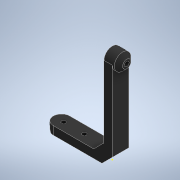
# Autodesk Inventor part: LinearActuatorToBottomPlateAdapter
Saved by Autodesk Inventor 2021 (Build 250183000, 183)
## iProperties
Created: 2020-07-16
Part Number: LinearActuatorToBottomPlateAdapter
Material: Generic
Document SubType Name: Modeling
Designer: CASE-SMALL2
Density: 1 g/cm^3
Appearance: Default
Author: CASE-SMALL2
## iProperties of the stored document _3DPrint.ipt
Created: 2020-07-17
Part Number: _3DPrint
Material: Generic
Document SubType Name: Modeling
Designer: CASE-SMALL2
Density: 1 g/cm^3
Appearance: Default
Author: CASE-SMALL2
Autodesk Inventor part; units mm, degrees
ref_plane "YZ Plane" through (0, 0, 0) normal (1, 0, 0) x (0, 1, 0)
ref_plane "XZ Plane" through (0, 0, 0) normal (0, 1, 0) x (-1, 0, 0)
ref_plane "XY Plane" through (0, 0, 0) normal (0, 0, 1) x (1, 0, 0)
sketch "Sketch3" plane through (0, 0, 0) normal (0, 0, 1) x (1, 0, 0)
  line L0 (0, 0) -> (65, 0)
  line L1 (65, 0) -> (65, 95)
  line L2 (65, 95) -> (57, 95)
  line L3 (57, 95) -> (57, 8)
  line L4 (57, 8) -> (0, 8)
  line L5 (0, 8) -> (0, 0)
  dimension "d17" = 8
  dimension "d18" = 57
  dimension "d19" = 87
  dimension "d20" = 8
  constraints: 12 end point, 5 perpendicular, 1 horizontal
  measures "d17" distance between parallel lines of L4 L0
  measures "d18" distance between parallel lines of L3 L5
  measures "d19" distance between parallel lines of L2 L4
  measures "d20" distance between parallel lines of L3 L1
extrude "Extrusion3" add sketch "Sketch3" against normal mid plane 16
sketch "Sketch5" plane through (0, 8, -8) normal (0, 1, 0) x (1, 0, 0)
  line L0 (-13, -8) -> (78, -8) projected
  circle A0 centre (10, -8) radius 1.9
  circle A1 centre (30, -8) radius 1.9
  line L1 (0, 0) -> (0, -16) projected
  point P0 (0, -8)
  dimension "d23" = 3.8
  dimension "d24" = 3.8
  dimension "d25" = 10
  dimension "d26" = 20
  constraints: 2 centre point, 2 point on line
  measures "d23" diameter of A0
  measures "d24" diameter of A1
  measures "d25" distance from line of L1 A0.centre
  measures "d26" distance of A0.centre A1.centre
extrude "Extrusion4" cut sketch "Sketch5" against normal through all
chamfer "Chamfer2" distance 5 angle 45 1 edges at (0, 0, 0)
chamfer "Chamfer3" distance 10 angle 45 1 edges at (57, 8, 0)
chamfer "Chamfer4" distance 10 angle 45 1 edges at (65, 0, 0)
sketch "Sketch6" plane through (65, 95, 8) normal (1, 0, 0) x (0, 0, -1)
  line L0 (16, -77) -> (16, 0) projected
  line L1 (0, -85) -> (0, 0) projected
  circle A0 centre (8, -8) radius 8
  line L2 (16, 0) -> (0, 0) projected
  point P0 (8, -95)
  dimension "d39" = 16
  constraints: 3 tangent, 1 centre point
  measures "d39" distance between parallel lines of L1 L0
extrude "Extrusion5" add sketch "Sketch6" along normal blind 7 contours A0
fillet "Fillet1" radius 8 2 edges at (61, 95, -8) (61, 95, 8)
sketch "Sketch7" plane through (57, 18, -8) normal (-1, 0, 0) x (0, 0, 1)
  point P0 (8, -18)
sketch "Sketch8" plane through (72, 87, 0) normal (1, 0, 0) x (0, 0, -1)
  circle A0 centre (0, 0) radius 8 projected
  circle A1 centre (0, 0) radius 2.75
  point P0 (0, -87)
  dimension "d43" = 5.5
  constraints: 1 centre point, 1 coincident
  measures "d43" diameter of A1
extrude "Extrusion6" add sketch "Sketch8" along normal blind 4 contours A1
sketch "Sketch9" plane through (76, 87, 0) normal (1, 0, 0) x (0, 0, -1)
  circle A0 centre (0, 0) radius 2.75 construction
  circle A1 centre (0, 0) radius 2.25
  point P0 (0, -87)
  dimension "d46" = 4.5
  constraints: 1 centre point
  measures "d46" diameter of A1
extrude "Extrusion7" cut sketch "Sketch9" against normal through all
sketch "Sketch10" plane through (57, 18, -8) normal (-1, 0, 0) x (0, 0, 1)
  circle A0 centre (8, 69) radius 2.25 projected
  circle A1 centre (8, 69) radius 4.5
  point P0 (8, -18)
  dimension "d49" = 9
  constraints: 1 centre point
  measures "d49" diameter of A1
extrude "Extrusion8" cut sketch "Sketch10" against normal blind 3
chamfer "Chamfer5" distance 3 angle 45 1 edges at (57, 87, -4.5)
chamfer "Chamfer6" distance 3 angle 45 1 edges at (72, 87, 2.75)
fillet "Fillet2" radius 8 2 edges at (0, 6.5, -8) (0, 6.5, 8)
sketch "Sketch11" plane through (76, 87, 0) normal (1, 0, 0) x (0, 0, -1)
  circle A0 centre (0, 0) radius 2.25 projected
  circle A1 centre (0, 0) radius 2.75 projected
  circle A2 centre (0, 0) radius 10.0452
  point P0 (0, -87)
  constraints: 1 centre point, 1 coincident
extrude "Extrusion9" cut sketch "Sketch11" against normal blind 5 contours A0 | A1 | A2
chamfer "Chamfer7" distance 4 angle 45 1 edges at (71, 87, 8)
equation "\"d20\" = d17"
body "Solid2"
